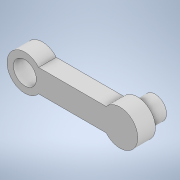
# Autodesk Inventor part: Component32
Saved by Autodesk Inventor 2022 (Build 260153000, 153)
## iProperties
Created: 2022-01-29
Part Number: Component32
Material: Generic
Document SubType Name: Modeling
Designer: Administrator
Density: 1 g/cm^3
Appearance: Default
Title: Component32
Author: Administrator
Autodesk Inventor part; units mm, degrees
ref_plane "YZ Plane" through (0, 0, 0) normal (1, 0, 0) x (0, 1, 0)
ref_plane "XZ Plane" through (0, 0, 0) normal (0, 1, 0) x (-1, 0, 0)
ref_plane "XY Plane" through (0, 0, 0) normal (0, 0, 1) x (1, 0, 0)
sketch "Sketch2" plane through (0, 0, 0) normal (0, 0, 1) x (1, 0, 0)
  arc A0 (-12.9361, 3.25) -> (-12.9361, -3.25) centre (-16.8404, 0) ccw
  line L0 (-12.9361, 3.25) -> (6.2552, 3.25)
  arc A1 (6.2552, -3.25) -> (6.2552, 3.25) centre (10.1596, 0) ccw
  circle A2 centre (10.1596, 0) radius 3.25
  line L1 (-12.9361, 3.25) -> (6.2552, 3.25)
  line L2 (6.2552, 3.25) -> (-12.9361, 3.25)
  arc A3 (-12.9361, 3.25) -> (-12.9361, -3.25) centre (-16.8404, 0) ccw
  arc A4 (-12.9361, 3.25) -> (-12.9361, -3.25) centre (-16.8404, 0) ccw
  circle A5 centre (-16.8404, 0) radius 3.25
  line L3 (-32.8836, 0) -> (22.6789, 0) construction
  line L4 (-12.9361, -3.25) -> (6.2552, -3.25)
  point P0 (0, 0)
  dimension "d8" = 27
  dimension "d9" = 6.5
  dimension "d10" = 6.5
  constraints: 10 end point, 8 point on circle, 6 centre point, 2 coincident, 2 equal radius, 2 point on line, 2 symmetric about line, 1 collinear, 1 horizontal, 1 parallel
  measures "d8" distance of A1.centre A0.centre
  measures "d9" distance between parallel lines of L4 L0
  measures "d10" diameter of A5
extrude "Extrusion3" add sketch "Sketch2" along normal blind 5 contours L0 A1 L4 A0 | A2
extrude "Extrusion4" add sketch "Sketch2" against normal blind 5 contours A2
equation "\"d9\" = width"
equation "\"d10\" = R"
equation "\"d4\" = thickness"
equation "\"d6\" = thickness"
equation "\"R\" = 6.5"
equation "\"thickness\" = 5"
equation "\"width\" = 6.5"
equation "\"R1\" = 9"
body "Solid2"
